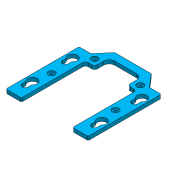
# Autodesk Inventor part: 16_035_BATTERY_HOLDER_BACK_R1
Saved by Autodesk Inventor 2021.2 (Build 252289000, 289)
## iProperties
Created: 2018-08-19
Part Number: 16_035_BATTERY_HOLDER_BACK_R1
Material: 一般
Document SubType Name: Modeling
Designer: y6tada
Density: 1 g/cm^3
Appearance: スカイ ブルー 標準
Mass: 1.43064 g
Surface Area: 22.0559 cm^2
Volume: 1.43064 cm^3
Author: y6tada
Autodesk Inventor part; units mm, degrees
ref_plane "YZ Plane" through (0, 0, 0) normal (1, 0, 0) x (0, 1, 0)
ref_plane "XZ Plane" through (0, 0, 0) normal (0, 1, 0) x (-1, 0, 0)
ref_plane "XY Plane" through (0, 0, 0) normal (0, 0, 1) x (1, 0, 0)
sketch "スケッチ1" plane through (0, 0, 0) normal (0, 0, 1) x (1, 0, 0)
  line L0 (0, 0) -> (0, 51.1276) construction
  line L1 (-6, 43) -> (6, 43) construction
  arc A0 (9, 40) -> (6, 43) centre (6, 40) ccw projected
  line L2 (9, 40) -> (9, 36.5) projected
  line L3 (10.5, 35) -> (12.5, 35)
  arc A1 (14, 33.5) -> (12.5, 35) centre (12.5, 33.5) ccw
  line L4 (14, 0) -> (14, 33.5) construction
  line L5 (10, 47) -> (-10, 47) construction
  line L6 (16, 40) -> (10, 47) construction
  line L7 (16, 26.6395) -> (16, 40) construction
  circle A2 centre (12.5, 38.5) radius 1.5 construction
  circle A3 centre (17.5, 20) radius 1.5 construction
  line L8 (22.5, 39.5) -> (22.5, 0.5)
  line L9 (22, 0) -> (14.5, 0)
  arc A4 (20.6, 30.9506) -> (17.4, 30.9506) centre (19, 33) ccw
  arc A5 (17.4, 29) -> (20.6, 29) centre (19, 29) ccw
  line L10 (17.4, 30.9506) -> (17.4, 29)
  line L11 (20.6, 30.9506) -> (20.6, 29)
  line L12 (19, 29) -> (19, 33) construction
  line L13 (10, 47) -> (16, 40)
  arc A6 (17.4, 7) -> (20.6, 7) centre (19, 7) ccw
  line L14 (17.4, 7) -> (17.4, 8.9506)
  line L15 (20.6, 7) -> (20.6, 8.9506)
  arc A7 (20.6, 8.9506) -> (17.4, 8.9506) centre (19, 11) ccw
  line L16 (19, 11) -> (19, 7) construction
  line L17 (14, 33.5) -> (14, 0.5)
  line L18 (0, 43) -> (0, 47)
  line L19 (0, 47) -> (10, 47)
  line L20 (6, 43) -> (0, 43)
  line L21 (16, 40) -> (22, 40)
  line L22 (22, 40) -> (22.5, 39.5)
  line L23 (22, 0) -> (22.5, 0.5)
  circle A8 centre (17.5, 20) radius 1.05
  circle A9 centre (12.5, 38.5) radius 1.05
  arc A10 (9, 36.5) -> (10.5, 35) centre (10.5, 36.5) ccw
  line L24 (14, 0.5) -> (14.5, 0)
  point P0 (22.5, 40)
  point P1 (22.5, 0)
  dimension "d5" = 2.6
  dimension "d6" = 4
  dimension "d10" = 4
  dimension "d14" = 0.5
  dimension "d15" = 0.5
  dimension "d17" = 0.5
  dimension "d18" = 0.5
  dimension "d19" = 2.1
  dimension "d20" = 9
  dimension "d21" = 9
  dimension "d22" = 2.1
  dimension "d23" = 1.5
  dimension "d24" = 1.6
  dimension "d25" = 2.6
  dimension "d26" = 1.6
  dimension "d28" = 38
  dimension "d29" = 45
  dimension "d30" = 40
  dimension "d31" = 0.5
  dimension "d32" = 0.5
  dimension "d36" = 28
  dimension "d37" = 10
  dimension "d38" = 6
  dimension "d39" = 7
  constraints: 38 end point, 12 point on circle, 9 vertical, 8 centre point, 8 tangent, 7 point on line, 5 collinear, 3 horizontal, 2 coincident, 2 midpoint, 1 equal radius
  measures "d5" radius of A4
  measures "d6" distance of L12.start L12.end
  measures "d10" distance of L16.start L16.end
  measures "d14" distance of L21.end point (22.5, 40)
  measures "d15" distance of L8.start point (22.5, 40)
  measures "d17" distance of L9.start point (22.5, 0)
  measures "d18" distance of L8.end point (22.5, 0)
  measures "d19" diameter of A8
  measures "d20" vertical distance of A8.centre L12.start
  measures "d21" vertical distance of L16.start A3.centre
  measures "d22" diameter of A9
  measures "d23" radius of A10
  measures "d24" radius of A5
  measures "d25" radius of A7
  measures "d26" radius of A6
  measures "d28" diameter of L12 L0
  measures "d29" diameter of L8 L0
  measures "d30" distance between parallel lines of L9 L21
  measures "d31" distance of L17.end point (14, 0)
  measures "d32" distance of L9.end point (14, 0)
  measures "d36" diameter of L4 L0
  measures "d37" distance of L18.end L5.start
  measures "d38" horizontal distance of L6.start L5.start
  measures "d39" distance from line of L6.start L5
extrude "押し出し1" add sketch "スケッチ1" along normal blind 2
sketch "スケッチ3" plane through (0, 0, 2) normal (0, 0, 1) x (1, 0, 0)
  circle A0 centre (17.5, 20) radius 1.05 projected
  circle A1 centre (17.5, 20) radius 1.8
  circle A2 centre (12.5, 38.5) radius 1.05 projected
  circle A3 centre (12.5, 38.5) radius 1.8
  point P0 (0, 0)
  dimension "d33" = 3.6
  constraints: 2 centre point, 2 coincident, 1 equal radius
  measures "d33" diameter of A3
extrude "押し出し2" cut sketch "スケッチ3" against normal blind 0.8
mirror "ミラー1" about plane through (0, 0, 0) normal (1, 0, 0) of "押し出し1", "押し出し2"
equation "\"d15\" = d14"
equation "\"d18\" = d17"
